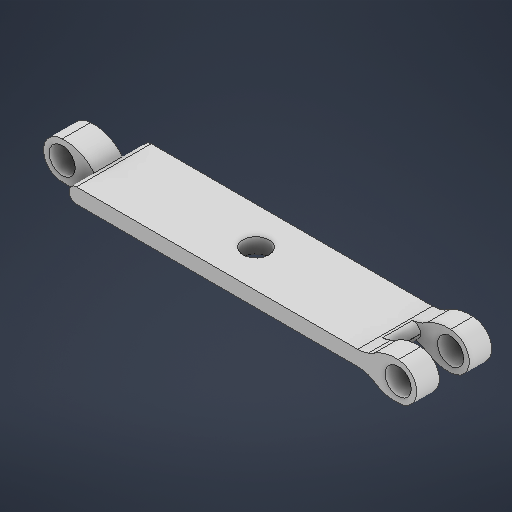
# Autodesk Inventor part: lamp_link
Saved by Autodesk Inventor 2027 (Build 310192060, 192F)
## iProperties
Created: 2026-05-15
Part Number: lamp_link
Material: Ogólny
Document SubType Name: Modeling
Designer: User
Density: 1 g/cm^3
Appearance: Domyślna
Author: User
Autodesk Inventor part; units mm, degrees
ref_plane "YZ Plane" through (0, 0, 0) normal (1, 0, 0) x (0, 1, 0)
ref_plane "XZ Plane" through (0, 0, 0) normal (0, 1, 0) x (-1, 0, 0)
sketch "Szkic1" plane through (0, 0, 0) normal (0, 1, 0) x (-1, 0, 0)
  line L0 (-20, 5) -> (20, 5)
  line L1 (20, 5) -> (20, -5)
  line L2 (20, -5) -> (-20, -5)
  line L3 (-20, -5) -> (-20, 5)
  line L4 (-20, 5) -> (20, -5) construction
  line L5 (20, 5) -> (-20, -5) construction
  point P0 (0, 0)
  dimension "d0" = 40
  dimension "d1" = 10
  constraints: 12 end point, 2 midpoint, 2 parallel, 1 horizontal, 1 perpendicular
  measures "d0" distance of L1.end L2.end
  measures "d1" distance of L0.end L1.end
extrude "Wyciągnięcie proste1" add sketch "Szkic1" along normal blind 2
sketch "Szkic2" plane through (-20, 0, 5) normal (0, 0, 1) x (1, 0, 0)
  line L0 (40, 0) -> (40, 2)
  line L1 (40, 1) -> (44, 1)
  line L2 (40, 1) -> (44, 1) construction
  circle A0 centre (44, 1) radius 1.75
  circle A1 centre (44, 1) radius 2.5
  line L3 (44, 3.5) -> (44, 3.5)
  line L4 (44, -1.5) -> (44, -1.5)
  arc A2 (44, 3.5) -> (40, 2) centre (43.5874, -1.4829) ccw
  arc A3 (40, 0) -> (44, -1.5) centre (43.5874, 3.4829) ccw
  line L5 (40, 2) -> (0, 2) projected
  line L6 (40, 0) -> (40, 2) projected
  line L7 (40, 2) -> (40, 0)
  line L8 (40, 2) -> (40, 0)
  line L9 (40, 1) -> (41.9498, 1)
  point P0 (20, 0)
  point P1 (44, 3.5)
  dimension "d4" = 4
  dimension "d5" = 0
  dimension "d6" = 3.5
  dimension "d7" = 5
  dimension "d8" = 0
  dimension "d9" = 0
  dimension "d10" = 5
  dimension "d11" = 5
  constraints: 16 end point, 6 point on circle, 4 centre point, 3 horizontal, 3 vertical, 2 coincident, 2 collinear, 2 midpoint
  measures "d4" distance of L1.start L1.end
  measures "d5" distance between parallel lines of L1 L2
  measures "d6" diameter of A0
  measures "d7" diameter of A1
  measures "d8" distance of L3.start L3.end
  measures "d9" distance of L4.start L4.end
  measures "d10" radius of A2
  measures "d11" radius of A3
extrude "Wyciągnięcie proste2" add sketch "Szkic2" against normal blind 3
ref_plane "Płaszczyzna konstrukcyjna1" through (-20, 0, 0) normal (0, 0, 1) x (1, 0, 0)
mirror "Odbij1" about plane through (-20, 0, 0) normal (0, 0, 1) of "Wyciągnięcie proste2"
sketch "Szkic3" plane through (-20, 0, 0) normal (0, 0, 1) x (1, 0, 0)
  line L0 (0, 0) -> (0, 2) projected
  line L1 (0, 2) -> (0, 0)
  line L2 (0, 2) -> (0, 0)
  line L3 (0, 1) -> (-4, 1)
  line L4 (0, 1) -> (-4, 1) construction
  circle A0 centre (-4, 1) radius 1.75
  circle A1 centre (-4, 1) radius 2.5
  line L5 (-4, -1.5) -> (-4, -1.5)
  line L6 (-4, 3.5) -> (-4, 3.5)
  arc A2 (-4, -1.5) -> (0, 0) centre (-3.5874, 3.4829) ccw
  arc A3 (0, 2) -> (-4, 3.5) centre (-3.5874, -1.4829) ccw
  line L7 (0, 1) -> (-2.4782, 1)
  point P0 (20, 0)
  point P1 (-4, -1.5)
  point P2 (-4, 3.5)
  dimension "d16" = 4
  dimension "d17" = 0
  dimension "d18" = 3.5
  dimension "d19" = 5
  dimension "d20" = 0
  dimension "d21" = 0
  dimension "d22" = 5
  dimension "d23" = 5
  constraints: 14 end point, 6 point on circle, 4 centre point, 2 coincident, 2 midpoint, 1 collinear, 1 horizontal, 1 vertical
  measures "d16" distance of L3.start L3.end
  measures "d17" distance between parallel lines of L3 L4
  measures "d18" diameter of A0
  measures "d19" diameter of A1
  measures "d20" distance of L5.start L5.end
  measures "d21" distance of L6.start L6.end
  measures "d22" radius of A2
  measures "d23" radius of A3
extrude "Wyciągnięcie proste3" add sketch "Szkic3" along normal mid plane 3.8
fillet "Zaokrąglenie1" radius 4 4 edges at (20, 2, -3.5) (20, 2, 3.5) (20, 0, -3.5) (20, 0, 3.5)
fillet "Zaokrąglenie2" radius 1 2 edges at (20, 2.258, 0) (20, -0.258, 0)
fillet "Zaokrąglenie3" radius 1 4 edges at (-20, 0, 3.45) (-20, 2, 3.45) (-20, 0, -3.45) (-20, 2, -3.45)
sketch "Szkic4" plane through (0, 2, 0) normal (0, 1, 0) x (1, 0, 0)
  line L0 (-19, 5) -> (-19, -5) projected
  line L1 (-19, 0) -> (18.5868, 0)
  line L2 (18.5868, 5) -> (18.5868, -5) projected
  circle A0 centre (0, 0) radius 1.75
  dimension "d29" = 3.5
  constraints: 2 end point, 2 midpoint, 1 centre point, 1 coincident
  measures "d29" diameter of A0
extrude "Wyciągnięcie proste4" cut sketch "Szkic4" against normal blind 10
